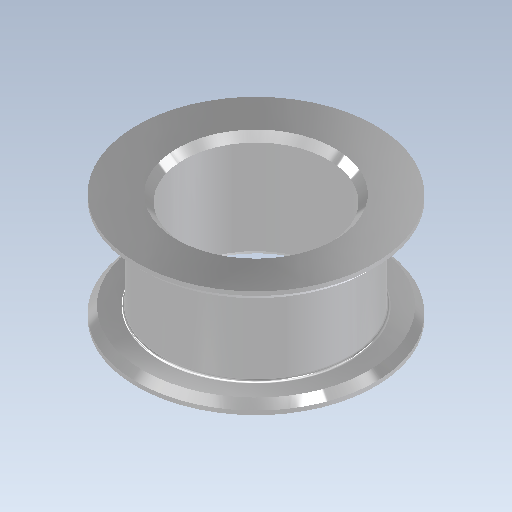
# Autodesk Inventor part: PoliaLisaGT2
Saved by Autodesk Inventor 2020 (Build 240168000, 168)
## iProperties
Created: 2014-01-28
Part Number: PoliaLisaGT2
Material: Aluminum 6061
Document SubType Name: Modeling
Designer: Fernando
Density: 2.7 g/cm^3
Appearance: Aluminum - Flat
Vendor: Ø20x12
Engineer: Fernando
Mass: 1.68206 g
Surface Area: 11.1587 cm^2
Volume: 0.622984 cm^3
Category: Impressora 3D
Manager: Fernando
Company: CNC Brasil
Author: Fernando
Title: Polia lisa
Autodesk Inventor part; units mm, degrees
ref_plane "YZ Plane" through (0, 0, 0) normal (1, 0, 0) x (0, 1, 0)
ref_plane "XZ Plane" through (0, 0, 0) normal (0, 1, 0) x (-1, 0, 0)
ref_plane "XY Plane" through (0, 0, 0) normal (0, 0, 1) x (1, 0, 0)
sketch "Esboço1" plane through (0, 0, 0) normal (1, 0, 0) x (0, 1, 0)
  line L0 (-4.05, 9) -> (-3.25, 9)
  line L1 (-3.25, 9) -> (-3.25, 7)
  line L2 (-3.25, 7) -> (3.25, 7)
  line L3 (3.25, 7) -> (3.25, 9)
  line L4 (3.25, 9) -> (4.05, 9)
  line L5 (4.05, 9) -> (4.05, 5.475)
  line L6 (-2.5, 5.475) -> (-4.05, 5.475)
  line L7 (-4.05, 5.475) -> (-4.05, 9)
  line L8 (-21.75, 0) -> (21.75, 0)
  line L9 (-2.5, 5.475) -> (-2.5, 5.475)
  line L10 (2.5, 5.475) -> (2.5, 5.475)
  line L11 (2.5, 5.475) -> (3.5, 5.475)
  line L12 (3.5, 5.475) -> (3.5, 5.475)
  line L13 (4.05, 5.475) -> (3.5, 5.475)
  line L14 (2.5, 5.475) -> (-2.5, 5.475)
  point P0 (0, 0)
  point P1 (0, 0)
  point P2 (0, 5.475)
  point P3 (0, 7)
  dimension "d3" = 0.8
  dimension "d4" = 14
  dimension "d5" = 18
  dimension "d11" = 2.5
  dimension "d14" = 10.95
  dimension "d16" = 6.5
  dimension "d17" = 2.5
  dimension "d19" = 10.95
  dimension "d20" = 125
  dimension "d21" = 0
  dimension "d22" = 1
  constraints: 30 end point, 7 parallel, 5 perpendicular, 2 equal length, 2 midpoint, 2 vertical alignment, 1 coincident, 1 collinear, 1 horizontal, 1 horizontal alignment, 1 point on line, 1 vertical
  measures "d3" distance of L0.start L0.end
  measures "d4" diameter of L2 L8
  measures "d5" diameter of L0 L8
  measures "d11" distance of L9.start point (0, 5.475)
  measures "d14" diameter of L6 L8
  measures "d16" distance between parallel lines of L3 L1
  measures "d17" distance from line of L10 point (0, 5.475)
  measures "d19" diameter of L14 L8
  measures "d20" angle of L14 L9
  measures "d21" distance between parallel lines of L14 L11
  measures "d22" distance between parallel lines of L10 L12
revolve "Revolução1" add sketch "Esboço1" angle 360 about axis through (0, -21.75, 0) along (0, 1, 0)
fillet "Arredondamento1" radius 0.2 2 edges at (0, 3.25, -7) (0, -3.25, -7)
chamfer "Chamfer2" distance 0.5 angle 45 2 edges at (0, -3.25, -9) (0, 3.25, -9)
chamfer "Chamfer3" distance 0.5 angle 45 2 edges at (0, -4.05, -5.475) (0, 4.05, -5.475)
